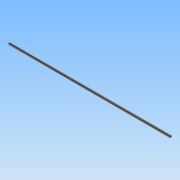
# Autodesk Inventor part: ВАЛ 5мм
Saved by Autodesk Inventor 2017 (Build 210142000, 142)
## iProperties
Part Number: ВАЛ 5мм
Material: Типовые
Document SubType Name: Modeling
Designer: Max
Mass: 7.12382 g
Surface Area: 57.3141 cm^2
Volume: 7.12382 cm^3
Density: 1 g/cm^3
Appearance: Сталь — полированная
Author: Max
Autodesk Inventor part; units mm, degrees
ref_plane "YZ Plane" through (0, 0, 0) normal (1, 0, 0) x (0, 1, 0)
ref_plane "XZ Plane" through (0, 0, 0) normal (0, 1, 0) x (-1, 0, 0)
ref_plane "XY Plane" through (0, 0, 0) normal (0, 0, 1) x (1, 0, 0)
sketch "Эскиз1" plane through (0, 0, 0) normal (1, 0, 0) x (0, 1, 0)
  circle A0 centre (0, 0) radius 2.5
  dimension "d0" = 5
  constraints: 1 centre point, 1 coincident
  measures "d0" diameter of A0
extrude "Выдавливание1" add sketch "Эскиз1" along normal mid plane 363
chamfer "Фаска1" distance 0.5 angle 45 2 edges at (181.5, -2.5, 0) (-181.5, -2.5, 0)
